Autodesk Inventor part; units mm, degrees
(part 2 of 2)
extrude "Extrusion14" add sketch "Sketch14" along normal blind 1.27 contours L0 S0 S1 S2 L1 L2 L3 S3 L4 S4 S5 L5 L6 S6 L7 L8 L9 L10 L11 L12 L13 S7 L14 L15 S8 S9 S10 L16 L17 S11 S12 L18 S13 S14 L19 S15 L20 L21 L22 L23 L24 S16 L25 L26 L27 S17 L28 L29 S18 L30 S19 S20 S21 S22 L31 S23 S24 S25 S26 S27 L32 L33 S28 L34 S29 L35 L36 | L56 L57 L58 L59 | L60 L61 S44 S45 L62 S93 S92 L85 L86 S59 S60 S61 S62 S63 L87 L75 S53 S54 S55 L76 | S93 S94 L118 S95 S96 S97 L119 S98 S99 L120 L121 L122 S100 L123 L88 S64 L89 S65 S66 L90 S67 S68 S69 S70 L91 S71 S72 S135 L174 L173 L172 L92 S73 L93 L94 L95 L96 S74 S75 L97 L98 L99 L100 S76 L101 L102 L103 S77 S78 S79 L104 L105 L106 L107 L108 L109 S80 S81 L110 S82 L111 S83 S84 S85 L112 S86 S87 L113 L114 S88 S89 L62 | L62 S89 S90 L115 L85 S92 S93 | S92 L87 S91 L116 L75 | L75 L116 L117 S92 | L62 S46 L63 L64 L65 L66 S47 L67 L68 S48 S49 L69 L70 S50 S51 L71 L72 L73 S52 L74 L75 L116 S91 L87 L77 S56 L78 L79 L80 S57 L81 L82 L115 L84 L85 S90 S89 | S92 L82 L115 S91 L87 | L85 L115 L84 S58 S92 | S92 S58 L84 L115 L82 | L82 L83 S58 S92 | S135 S136 L175 L176 L177 S137 L178 L179 L180 L181 S138 S139 L182 L183 S101 S102 S103 L124 S104 S105 S106 L125 S107 L126 L127 L128 L129 L130 L131 L132 L133 L134 L135 L136 S108 L137 L138 L139 L140 S109 L141 S110 S111 S112 S113 S114 S115 S116 L142 S117 L143 L144 S118 S119 S120 L145 L146 L147 L148 L149 L150 L151 S121 L152 L153 S122 L154 L155 L156 S157 S124 L158 L159 S125 S126 L160 S127 L161 L162 S128 L163 L164 L165 L166 S129 L167 S130 S131 L168 L169 L170 L171 S132 S133 S134 L172 S72 | S72 L172 L173 L174 S135 | S157 L156 S153 S154 S124 | S124 S154 L201 L202 L203 L204 S155 L205 L206 S156 L207 L208 L209 S157 | S154 S153 L156 S123 L157 S124 | S157 S158 L210 S159 L211 L212 L213 L214 L215 L216 L217 L218 S160 S161 S162 L219 S163 L220 S164 L221 S165 S166 S167 L222 L223 S168 L224 S169 L225 L226 L227 S170 L228 L229 S171 L230 L231 L232 L233 L234 L235 S172 L236 L237 L238 L239 S173 S140 S210 L274 L273 L272 S209 S141 L184 S142 L185 S203 S143 S144 S145 L187 L188 L189 L190 L191 L192 L193 S146 L194 L195 S147 S148 S149 L196 L197 L198 S150 S202 L269 L268 S151 S152 S153 L156 | L268 L269 S202 S150 L267 S201 L200 S151 | S151 L200 S201 L268 | S201 L267 S150 L199 L200 | S202 S203 S143 L186 S199 S200 L267 S150 | S203 L185 S199 L186 S143 | S203 S204 L270 S205 S206 S207 L271 S208 S209 S140 S210 L275 L240 S174 L241 S175 S176 L242 S177 S178 S179 S180 L243 S181 S182 L244 S183 L245 L246 L247 L248 S184 S185 L249 L250 L251 L252 S186 L253 L254 L255 S187 S188 S189 L256 L257 L258 L259 L260 L261 S190 S191 L262 S192 L263 S193 S194 S195 L264 S196 S197 L265 L266 S198 S199 L185 | S199 L185 L186 | S209 L272 L273 L274 S210 S140
ref_plane "Work Plane2" through (-162.56, -10.16, 33.845) normal (0, 0, 1) x (1, 0, 0)
sketch "Sketch16" plane through (-162.56, -10.16, 33.845) normal (0, 0, 1) x (1, 0, 0)
  line L0 (172.72, 27.182) -> (0, 27.182) projected
  line L1 (0, 27.182) -> (0, -51.918) projected
  line L2 (0, -51.918) -> (5.08, -51.918) projected
  line L3 (5.08, -51.918) -> (79.6753, -14.29) projected
  line L4 (70.0258, -5.5057) -> (69.9518, -4.1001) projected
  line L5 (75.3154, 2.6321) -> (75.4264, 2.3362) projected
  line L6 (75.2045, 1.4484) -> (75.2045, 1.2635) projected
  line L7 (75.2045, 1.2635) -> (75.3154, 1.2635) projected
  line L8 (75.3154, 1.2635) -> (75.2045, -0.697) projected
  line L9 (75.2045, -0.697) -> (75.2045, -1.1779) projected
  line L10 (75.2045, -1.1779) -> (75.7223, -3.5453) projected
  line L11 (75.7223, -3.5453) -> (75.4264, -3.8412) projected
  line L12 (75.4264, -3.8412) -> (75.2045, -3.8412) projected
  line L13 (75.2045, -3.8412) -> (75.1305, -3.7302) projected
  line L14 (75.1305, -3.7302) -> (75.0195, -3.7302) projected
  line L15 (75.0195, -3.7302) -> (75.1305, -3.6192) projected
  line L16 (75.1305, -3.6192) -> (75.1305, -3.5453) projected
  line L17 (74.0578, -2.1766) -> (73.6509, -2.1766) projected
  line L18 (73.6509, -2.1766) -> (73.281, -2.2876) projected
  line L19 (73.281, -2.2876) -> (73.17, -2.1766) projected
  line L20 (73.17, -2.1766) -> (73.059, -2.1766) projected
  line L21 (71.4314, -4.2111) -> (71.4314, -4.9139) projected
  line L22 (78.4596, 8.1067) -> (78.3486, 8.1067) projected
  line L23 (73.6509, 10.622) -> (73.6509, 10.733) projected
  line L24 (73.6509, 10.733) -> (75.4264, 10.733) projected
  line L25 (61.0742, 20.7944) -> (59.5946, 21.0903) projected
  line L26 (59.5946, 21.0903) -> (59.1877, 20.9793) projected
  line L27 (59.1877, 20.9793) -> (58.1149, 21.2752) projected
  line L28 (58.1149, 21.2752) -> (57.819, 21.1643) projected
  line L29 (57.819, 21.1643) -> (57.2642, 21.2752) projected
  line L30 (57.2642, 21.2752) -> (57.1532, 21.1643) projected
  line L31 (57.1532, 21.1643) -> (57.0422, 21.1643) projected
  line L32 (52.9733, 21.8671) -> (52.5664, 21.7561) projected
  line L33 (52.5664, 21.7561) -> (52.2705, 21.8671) projected
  line L34 (49.5332, 21.3492) -> (49.4222, 21.4602) projected
  line L35 (49.4222, 21.4602) -> (49.3482, 21.4602) projected
  line L36 (49.3482, 21.4602) -> (46.9921, 20.7411) projected
  line L37 (57.1902, 17.0583) -> (57.2642, 16.9844) projected
  line L38 (57.856, 16.6884) -> (57.856, 16.7624) projected
  line L39 (57.856, 16.7624) -> (58.4479, 17.8351) projected
  line L40 (58.4479, 17.8351) -> (57.2642, 19.0188) projected
  line L41 (57.2642, 19.0188) -> (57.2642, 19.1298) projected
  line L42 (57.2642, 19.1298) -> (57.3751, 19.1298) projected
  line L43 (57.3751, 19.1298) -> (61.666, 17.1693) projected
  line L44 (61.666, 17.1693) -> (61.666, 16.8734) projected
  line L45 (61.666, 16.8734) -> (60.7782, 17.0583) projected
  line L46 (65.1801, 4.0747) -> (65.1801, 3.7788) projected
  line L47 (64.5882, 1.2635) -> (63.4046, 1.4484) projected
  line L48 (62.0359, 0.3757) -> (62.0359, 0.0798) projected
  line L49 (72.3932, 2.6321) -> (72.5042, 2.6321) projected
  line L50 (72.5042, 2.6321) -> (72.5042, 2.1143) projected
  line L51 (65.2911, -2.4725) -> (62.6647, -3.1384) projected
  line L52 (67.9174, -4.3221) -> (67.9174, -4.507) projected
  line L53 (67.9174, -4.507) -> (63.4046, -4.0261) projected
  line L54 (63.4046, -4.0261) -> (62.1469, -4.0261) projected
  line L55 (58.3369, -5.2098) -> (57.0792, -5.3948) projected
  line L56 (57.0792, -5.3948) -> (56.3024, -5.3948) projected
  line L57 (51.4197, -3.8412) -> (51.0128, -3.8412) projected
  line L58 (51.0128, -3.8412) -> (50.6429, -4.2111) projected
  line L59 (50.6429, -4.2111) -> (50.6429, -4.618) projected
  line L60 (50.6429, -4.618) -> (51.0128, -4.9879) projected
  line L61 (51.0128, -4.9879) -> (51.4197, -4.9879) projected
  line L62 (51.4197, -4.9879) -> (52.0115, -4.507) projected
  line L63 (58.3369, -8.428) -> (60.1864, -8.7239) projected
  line L64 (60.1864, -8.7239) -> (60.5933, -8.6129) projected
  line L65 (60.5933, -8.6129) -> (60.7043, -8.7239) projected
  line L66 (60.7043, -8.7239) -> (60.7043, -8.7979) projected
  line L67 (48.3125, -12.6079) -> (47.5357, -12.6819) projected
  line L68 (47.5357, -12.6819) -> (45.4643, -12.6819) projected
  line L69 (25.4525, -8.206) -> (23.9729, -8.0951) projected
  line L70 (24.7497, -2.7315) -> (24.7497, -3.9891) projected
  line L71 (35.5139, -2.1396) -> (32.1847, -3.3973) projected
  line L72 (21.5315, 4.9995) -> (20.9767, 6.738) projected
  line L73 (35.033, 18.8339) -> (35.144, 18.8339) projected
  line L74 (35.144, 18.8339) -> (29.7434, 15.2458) projected
  line L75 (29.7434, 15.2458) -> (29.7434, 15.1348) projected
  line L76 (29.7434, 15.1348) -> (30.1503, 15.2458) projected
  line L77 (37.1784, 14.7649) -> (35.5879, 16.6884) projected
  line L78 (35.5879, 16.6884) -> (35.5879, 16.7994) projected
  line L79 (35.5879, 16.7994) -> (41.5063, 12.2496) projected
  line L80 (41.5063, 12.2496) -> (41.4323, 12.2496) projected
  line L81 (40.2486, 12.6565) -> (39.3609, 12.6565) projected
  line L82 (39.3609, 12.6565) -> (37.7333, 10.696) projected
  line L83 (37.7333, 10.696) -> (37.7333, 10.622) projected
  line L84 (34.5891, 6.2942) -> (36.0317, 3.8528) projected
  line L85 (36.0317, 3.8528) -> (35.9578, 3.8528) projected
  line L86 (35.9578, 3.8528) -> (28.7816, 9.4753) projected
  line L87 (28.7816, 9.4753) -> (28.8556, 9.4753) projected
  line L88 (28.8556, 9.4753) -> (31.408, 8.4026) projected
  line L89 (31.408, 8.4026) -> (31.5189, 8.4026) projected
  line L90 (32.1108, 12.5085) -> (31.8888, 12.5085) projected
  line L91 (24.2688, 6.3681) -> (24.2688, 6.2572) projected
  line L92 (38.0662, -0.9559) -> (39.028, -0.9559) projected
  line L93 (40.5076, -2.3246) -> (40.5076, -2.4355) projected
  line L94 (40.5076, -2.4355) -> (40.5815, -2.4355) projected
  line L95 (48.3761, 2.6511) -> (48.3865, 2.7061) projected
  line L96 (48.3865, 2.7061) -> (48.4402, 2.7061) projected
  line L97 (51.5307, 6.1462) -> (54.3829, 11.2735) projected
  line L98 (53.0843, 11.9907) -> (53.1582, 12.1016) projected
  line L99 (53.1582, 12.1016) -> (54.7533, 12.1016) projected
  line L100 (56.0065, 13.7662) -> (56.0814, 13.7662) projected
  line L101 (43.9318, 19.8071) -> (43.6517, 19.7216) projected
  line L102 (40.0637, 18.6489) -> (40.0637, 18.8339) projected
  line L103 (38.991, 21.1643) -> (38.732, 21.0903) projected
  line L104 (38.732, 21.0903) -> (32.2587, 21.8671) projected
  line L105 (32.2587, 21.8671) -> (31.9628, 21.7561) projected
  line L106 (31.9628, 21.7561) -> (31.6669, 21.8671) projected
  line L107 (25.8964, 20.6834) -> (19.4601, 19.0188) projected
  line L108 (19.4601, 19.0188) -> (19.4601, 19.2038) projected
  line L109 (29.8174, 22.4589) -> (31.297, 22.6439) projected
  line L110 (31.297, 22.6439) -> (31.7779, 22.5329) projected
  line L111 (31.7779, 22.5329) -> (33.3314, 22.5329) projected
  line L112 (49.9401, 22.4589) -> (51.3827, 22.6439) projected
  line L113 (51.3827, 22.6439) -> (53.4542, 22.6439) projected
  line L114 (78.2377, 15.8007) -> (78.3486, 15.8007) projected
  line L115 (79.0514, 17.1693) -> (77.7568, 18.7229) projected
  line L116 (77.7568, 18.7229) -> (77.9787, 18.7229) projected
  line L117 (82.3436, 16.2815) -> (82.2696, 16.2076) projected
  line L118 (82.2696, 16.2076) -> (82.1586, 16.2076) projected
  line L119 (82.1586, 16.2076) -> (81.3818, 16.3925) projected
  line L120 (81.3818, 16.3925) -> (81.2709, 16.3925) projected
  line L121 (80.0132, 14.8389) -> (79.9022, 14.432) projected
  line L122 (85.4878, 2.0403) -> (85.4878, 1.7444) projected
  line L123 (85.4878, 1.7444) -> (85.2658, 0.0798) projected
  line L124 (85.2658, 0.0798) -> (84.711, 0.0798) projected
  line L125 (84.711, 0.0798) -> (84.6, 0.1908) projected
  line L126 (91.4432, 2.0403) -> (91.6141, 2.3631) projected
  line L127 (90.4075, 4.9995) -> (89.8526, 6.738) projected
  line L128 (103.9089, 18.8339) -> (104.0199, 18.8339) projected
  line L129 (104.0199, 18.8339) -> (98.6193, 15.2458) projected
  line L130 (98.6193, 15.2458) -> (98.6193, 15.1348) projected
  line L131 (98.6193, 15.1348) -> (99.0262, 15.2458) projected
  line L132 (106.0544, 14.7649) -> (104.4638, 16.6884) projected
  line L133 (104.4638, 16.6884) -> (104.4638, 16.7994) projected
  line L134 (104.4638, 16.7994) -> (110.3822, 12.2496) projected
  line L135 (110.3822, 12.2496) -> (110.3082, 12.2496) projected
  line L136 (109.1246, 12.6565) -> (108.2368, 12.6565) projected
  line L137 (108.2368, 12.6565) -> (106.6092, 10.696) projected
  line L138 (106.6092, 10.696) -> (106.6092, 10.622) projected
  line L139 (103.465, 6.2942) -> (104.9077, 3.8528) projected
  line L140 (104.9077, 3.8528) -> (104.8337, 3.8528) projected
  line L141 (104.8337, 3.8528) -> (97.6576, 9.4753) projected
  line L142 (97.6576, 9.4753) -> (97.7315, 9.4753) projected
  line L143 (97.7315, 9.4753) -> (100.2839, 8.4026) projected
  line L144 (100.2839, 8.4026) -> (100.3948, 8.4026) projected
  line L145 (100.9867, 12.5085) -> (100.7647, 12.5085) projected
  line L146 (93.1447, 6.3681) -> (93.1447, 6.2572) projected
  line L147 (106.9421, -0.9559) -> (107.9039, -0.9559) projected
  line L148 (109.3835, -2.3246) -> (109.3835, -2.4355) projected
  line L149 (109.3835, -2.4355) -> (109.4575, -2.4355) projected
  line L150 (116.6706, 2.1708) -> (116.6706, 7.5518) projected
  line L151 (114.895, 6.3681) -> (114.7101, 6.5901) projected
  line L152 (114.7101, 6.5901) -> (114.5251, 6.5901) projected
  line L153 (114.5251, 6.5901) -> (114.5251, 12.1386) projected
  line L154 (114.5251, 12.1386) -> (114.7101, 12.1386) projected
  line L155 (115.9678, 10.2891) -> (116.6706, 10.2891) projected
  line L156 (116.6706, 10.2891) -> (116.6706, 13.2113) projected
  line L157 (113.3414, 14.9869) -> (113.3414, 15.1718) projected
  line L158 (113.3414, 15.1718) -> (124.1796, 15.1718) projected
  line L159 (121.1464, 25.825) -> (121.0724, 26.3799) projected
  line L160 (121.0724, 26.3799) -> (121.1464, 26.4909) projected
  line L161 (121.1464, 26.4909) -> (121.2574, 26.4909) projected
  line L162 (124.8824, 16.2445) -> (124.9564, 15.5417) projected
  line L163 (124.9564, 15.5417) -> (124.9564, 13.7662) projected
  line L164 (124.9564, 13.7662) -> (124.9934, 13.7662) projected
  line L165 (124.9934, 13.7662) -> (124.9934, 13.6922) projected
  line L166 (124.9564, 13.6059) -> (124.9564, 13.5073) projected
  line L167 (124.8824, -8.6499) -> (124.8824, -8.8719) projected
  line L168 (124.8824, -8.8719) -> (112.7496, -8.8719) projected
  line L169 (112.7496, -8.8719) -> (112.7496, -8.7609) projected
  line L170 (116.6706, -4.1741) -> (116.6706, 0.9725) projected
  line L171 (100.9867, -8.391) -> (100.1729, -8.5759) projected
  line L172 (114.4512, -11.9051) -> (116.0047, -11.9051) projected
  line L173 (126.362, -8.9828) -> (127.5457, -8.6869) projected
  line L174 (127.5457, -8.6869) -> (127.6567, -8.7979) projected
  line L175 (127.6567, -8.7979) -> (127.6567, -8.8719) projected
  line L176 (117.1884, -12.6079) -> (116.4116, -12.6819) projected
  line L177 (116.4116, -12.6819) -> (114.3402, -12.6819) projected
  line L178 (94.3284, -8.206) -> (92.8488, -8.0951) projected
  line L179 (93.6256, -2.7315) -> (93.6256, -3.9891) projected
  line L180 (104.3898, -2.1396) -> (101.0607, -3.3973) projected
  line L181 (80.3091, -7.5402) -> (79.4213, -8.0211) projected
  line L182 (79.4213, -8.0211) -> (79.3104, -8.1321) projected
  line L183 (79.3104, -8.1321) -> (78.9405, -8.0211) projected
  line L184 (75.7223, -8.502) -> (75.4264, -8.428) projected
  line L185 (75.4264, -8.428) -> (74.9455, -8.502) projected
  line L186 (74.9455, -8.502) -> (74.3537, -8.502) projected
  line L187 (74.3537, -8.502) -> (73.8728, -8.428) projected
  line L188 (80.5857, -13.8307) -> (86.36, -10.918) projected
  line L189 (167.64, -51.918) -> (86.36, -10.918) projected
  line L190 (172.72, -51.918) -> (167.64, -51.918) projected
  line L191 (172.72, 27.182) -> (172.72, -51.918) projected
  line L192 (146.7807, 18.8709) -> (146.7807, 19.0928) projected
  line L193 (146.7807, 19.0928) -> (147.0766, 19.0928) projected
  line L194 (147.0766, 19.0928) -> (147.0766, 18.8709) projected
  line L195 (147.0766, 18.8709) -> (146.7807, 18.8709) projected
  line L196 (128.2115, -5.0619) -> (128.3225, -4.9509) projected
  line L197 (128.3225, -4.9509) -> (127.4347, -3.8782) projected
  line L198 (127.4347, -3.8782) -> (127.4347, -3.7672) projected
  line L199 (128.6924, -4.47) -> (128.9883, -4.47) projected
  line L200 (139.8265, 5.7023) -> (139.8265, 12.4345) projected
  line L201 (139.8265, 12.4345) -> (140.0484, 12.4345) projected
  line L202 (141.4911, 9.8082) -> (142.8597, 9.6233) projected
  line L203 (142.8597, 9.6233) -> (143.3406, 9.6233) projected
  line L204 (143.3406, 9.6233) -> (143.3406, 13.3223) projected
  line L205 (143.3406, 13.3223) -> (139.5306, 15.1718) projected
  line L206 (139.5306, 15.1718) -> (139.5306, 15.3568) projected
  line L207 (139.5306, 15.3568) -> (142.1939, 15.3568) projected
  line L208 (142.1939, 15.3568) -> (142.5638, 15.4678) projected
  line L209 (143.7475, 15.1718) -> (143.9324, 14.9869) projected
  line L210 (143.9324, 14.9869) -> (144.5243, 14.9869) projected
  line L211 (148.0383, 18.6859) -> (147.3725, 18.7599) projected
  line L212 (147.3725, 18.7599) -> (147.3725, 18.9818) projected
  line L213 (153.6239, 25.3072) -> (153.8088, 25.3072) projected
  line L214 (148.9261, 9.6233) -> (149.333, 9.6233) projected
  line L215 (150.8866, 9.9932) -> (151.3675, 12.0646) projected
  line L216 (151.3675, 12.0646) -> (151.5524, 12.0646) projected
  line L217 (151.5524, 12.0646) -> (151.5524, 4.4446) projected
  line L218 (151.5524, 4.4446) -> (151.3675, 4.4446) projected
  line L219 (151.3675, 4.4446) -> (151.3675, 4.8146) projected
  line L220 (150.1838, 6.4791) -> (147.5575, 6.4791) projected
  line L221 (147.5575, 6.4791) -> (147.5575, 5.7763) projected
  line L222 (147.5575, 5.7763) -> (147.6684, 2.8541) projected
  line L223 (147.4465, 2.2622) -> (147.5575, 0.8196) projected
  line L224 (147.5575, 0.8196) -> (147.5575, -2.1026) projected
  line L225 (146.1888, -2.6945) -> (145.8189, -3.5822) projected
  line L226 (155.9543, 6.2942) -> (156.1392, 6.2942) projected
  line L227 (132.9093, -8.391) -> (132.7983, -8.391) projected
  line L228 (132.7983, -8.391) -> (132.7983, -8.465) projected
  line L229 (134.2779, -9.7226) -> (136.9043, -11.3872) projected
  line L230 (140.2334, -12.5709) -> (140.2334, -12.6819) projected
  line L231 (140.2334, -12.6819) -> (139.4566, -12.9778) projected
  line L232 (139.4566, -12.9778) -> (139.0497, -12.9778) projected
  point P0 (162.56, 10.16)
  point P1 (72.8741, -9.9076)
  point P2 (71.2095, -7.8361)
  point P3 (71.0246, -1.7697)
  point P4 (73.281, 1.1525)
  point P5 (73.7618, -6.7634)
  point P6 (76.5731, -5.2838)
  point P7 (79.6063, -1.1779)
  point P8 (80.901, 4.1857)
  point P9 (78.4596, 11.6947)
  point P10 (77.6458, 9.6603)
  point P11 (76.98, 13.3593)
  point P12 (66.8077, 18.9448)
  point P13 (51.1978, 19.3147)
  point P14 (59.4096, 15.5047)
  point P15 (63.1456, 11.2139)
  point P16 (63.5155, -0.9929)
  point P17 (70.3587, 0.9676)
  point P18 (59.5206, -9.3897)
  point P19 (58.077, -9.1972)
  point P20 (19.608, -8.6869)
  point P21 (28.5967, -6.8374)
  point P22 (35.4029, -4.692)
  point P23 (36.6976, -3.3973)
  point P24 (25.1566, 0.1168)
  point P25 (35.5139, 12.6195)
  point P26 (42.2461, 2.928)
  point P27 (36.8455, 9.7343)
  point P28 (34.5151, 11.4358)
  point P29 (28.4857, 2.6321)
  point P30 (34.7371, 0.1908)
  point P31 (43.2079, 0.4127)
  point P32 (46.0561, 1.0785)
  point P33 (49.9771, 4.1117)
  point P34 (56.3764, 14.432)
  point P35 (48.8674, 18.242)
  point P36 (42.9844, 20.1106)
  point P37 (45.4891, 21.137)
  point P38 (73.6509, 18.0571)
  point P39 (82.7505, 11.3988)
  point P40 (83.0464, -1.2888)
  point P41 (84.3041, -2.8424)
  point P42 (104.3898, 12.6195)
  point P43 (111.122, 2.928)
  point P44 (105.7214, 9.7343)
  point P45 (103.3911, 11.4358)
  point P46 (97.3616, 2.6321)
  point P47 (103.613, 0.1908)
  point P48 (112.0838, 0.4127)
  point P49 (114.932, 1.0785)
  point P50 (113.9333, 14.7649)
  point P51 (122.626, 21.1273)
  point P52 (121.1464, -5.0619)
  point P53 (122.1451, -7.0223)
  point P54 (116.0787, -6.9114)
  point P55 (110.2713, -3.8042)
  point P56 (103.3911, -9.6487)
  point P57 (111.6399, -11.4242)
  point P58 (121.6643, -10.4624)
  point P59 (88.484, -8.6869)
  point P60 (97.4726, -6.8374)
  point P61 (104.2788, -4.692)
  point P62 (105.5735, -3.3973)
  point P63 (94.0325, 0.1168)
  point P64 (92.0716, 1.8529)
  point P65 (86.1536, -4.2111)
  point P66 (78.5336, -12.6079)
  point P67 (131.4297, -8.9458)
  point P68 (129.0993, -6.4305)
  point P69 (133.2792, 1.7074)
  point P70 (148.8151, 16.1336)
  point P71 (149.333, 17.6872)
  point P72 (151.7374, 17.5022)
  point P73 (152.5142, 16.4295)
  point P74 (147.1506, -4.8399)
  point P75 (150.1098, -3.2863)
  point P76 (154.4746, 1.1895)
  point P77 (154.4007, 0.2278)
  point P78 (151.3675, -3.3973)
  point P79 (147.4465, -6.6154)
  point P80 (136.4234, -8.7609)
  constraints: 174 other
sketch "Sketch17" plane through (-162.56, -10.16, 33.845) normal (0, 0, 1) x (1, 0, 0)
  line L0 (152.4, 27.182) -> (172.72, 27.182) projected
  line L1 (127.508, 27.182) -> (152.4, 27.182) projected
  line L2 (45.212, 27.182) -> (127.508, 27.182) projected
  line L3 (20.32, 27.182) -> (45.212, 27.182) projected
  line L4 (0, 27.182) -> (20.32, 27.182) projected
  line L5 (172.72, 27.182) -> (0, 27.182) projected
  line L6 (172.72, 27.182) -> (172.72, 24.642)
  line L7 (172.72, 19.132) -> (172.72, -2.868) projected
  line L8 (172.72, 24.642) -> (160.02, 24.642)
  line L9 (160.02, 24.642) -> (147.32, 24.642)
  line L10 (147.32, 24.642) -> (147.32, 20.832)
  line L11 (147.32, 20.832) -> (160.02, 20.832)
  line L12 (160.02, 20.832) -> (160.02, 24.642)
  line L13 (133.35, 24.642) -> (120.65, 24.642)
  line L14 (133.35, 20.832) -> (133.35, 24.642)
  line L15 (120.65, 20.832) -> (133.35, 20.832)
  line L16 (120.65, 24.642) -> (120.65, 20.832)
  line L17 (106.68, 24.642) -> (93.98, 24.642)
  line L18 (106.68, 20.832) -> (106.68, 24.642)
  line L19 (93.98, 20.832) -> (106.68, 20.832)
  line L20 (93.98, 24.642) -> (93.98, 20.832)
  line L21 (80.01, 24.642) -> (67.31, 24.642)
  line L22 (80.01, 20.832) -> (80.01, 24.642)
  line L23 (67.31, 20.832) -> (80.01, 20.832)
  line L24 (67.31, 24.642) -> (67.31, 20.832)
  line L25 (53.34, 24.642) -> (40.64, 24.642)
  line L26 (53.34, 20.832) -> (53.34, 24.642)
  line L27 (40.64, 20.832) -> (53.34, 20.832)
  line L28 (40.64, 24.642) -> (40.64, 20.832)
  line L29 (26.67, 24.642) -> (13.97, 24.642)
  line L30 (26.67, 20.832) -> (26.67, 24.642)
  line L31 (13.97, 20.832) -> (26.67, 20.832)
  line L32 (13.97, 24.642) -> (13.97, 20.832)
  point P0 (162.56, 10.16)
  dimension "d71" = 2.54
  dimension "d72" = 12.7
  dimension "d73" = 12.7
  dimension "d74" = 3.81
  dimension "d77" = 26.67
  constraints: 52 end point, 2 collinear, 2 horizontal, 2 parallel, 2 perpendicular, 39 other
  measures "d71" distance of L5.start L6.end
  measures "d72" distance of L6.end L8.end
  measures "d73" distance of L11.end L10.end
  measures "d74" distance of L10.end L9.end
  measures "d77" distance of L8.end L13.start
extrude "Extrusion16" cut sketch "Sketch17" against normal blind 254
body "Solid1"
